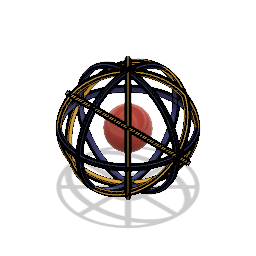
01-Atom v3 (Autodesk Fusion 360 design; units mm, degrees)
Autodesk Fusion 360 part; units mm, degrees
note: some values were not read from the file. Set by a fixed rule: which sketch regions a step uses.
sketch "Sketch1" plane through (0, 0, 0) normal (0, 1, 0) x (1, 0, 0)
  line L0 (1, 20) -> (1, 20.5)
  line L1 (-1, 20.5) -> (-1, 20)
  line L2 (-1, 20.5) -> (-0.9, 20.8)
  line L3 (0.9, 20.8) -> (1, 20.5)
  line L4 (-0.9, 20.8) -> (-0.95, 21.0122)
  line L5 (0.9, 20.8) -> (0.95, 21.0122)
  line L6 (-0.95, 21.0122) -> (-0.7, 21.5)
  line L7 (0.7, 21.5) -> (0.95, 21.0122)
  line L8 (-0.7, 21.5) -> (-0.4, 21.6)
  line L9 (0.4, 21.6) -> (0.7, 21.5)
  line L10 (-0.4, 21.6) -> (0, 21.65)
  line L11 (0, 21.65) -> (0.4, 21.6)
  arc A0 (1, 20) -> (-1, 20) centre (0, 15.0499) ccw
revolve "Revolve1" add sketch "Sketch1" angle 360 about axis through (1.75, 0, 0) along (1, 0, 0) makes body 1
copy_body "CopyPasteBodies1" bodies 1 makes body 2
move_body "Move1" bodies 2 to x (0, 0, -1) y (0, 1, 0) z (1, 0, 0) at (0, 0, 0)
copy_body "CopyPasteBodies2" bodies 2 makes body 3
move_body "Move2" bodies 3 to x (1, 0, 0) y (0, 0, -1) z (0, 1, 0) at (0, 0, 0)
copy_body "CopyPasteBodies3" bodies 2 makes body 4
move_body "Move3" bodies 4 1 to x (0.707107, 0, -0.707107) y (0, 1, 0) z (0.707107, 0, 0.707107) at (0, 0, 0)
copy_body "CopyPasteBodies4" bodies 2 makes body 5
move_body "Move4" bodies 5 to x (0, 0, -1) y (0, 1, 0) z (1, 0, 0) at (0, 0, 0)
copy_body "CopyPasteBodies5" bodies 3 makes body 6
move_body "Move5" bodies 6 to x (1, 0, 0) y (0, 0.707107, -0.707107) z (0, 0.707107, 0.707107) at (0, 0, 0)
copy_body "CopyPasteBodies6" bodies 3 makes body 7
move_body "Move6" bodies 7 to x (1, 0, 0) y (0, 0.707107, 0.707107) z (0, -0.707107, 0.707107) at (0, 0, 0)
sketch "Sketch2" plane through (0, 0, 0) normal (0, 1, 0) x (1, 0, 0)
  circle A0 centre (0, 0) radius 7.5
  line L0 (0, 7.5) -> (0, -7.5)
  dimension "d9" = 15
  constraint coincident A0.centre origin
  constraint coincident A0 L0.start
  constraint coincident A0 L0.end
  constraint vertical L0
  measures "d9" diameter of A0
revolve "Revolve2" add sketch "Sketch2" angle 360 about axis through (0, 0, -7.5) along (0, 0, 1) separate body contours A0 L0 picked at (2.6973, 1.9652) makes body 8
